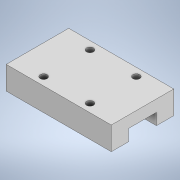
# Autodesk Inventor part: Linear_Rail_Carrier_Basic
Saved by Autodesk Inventor 2021 (Build 250183000, 183)
## iProperties
Created: 2021-03-29
Part Number: Linear_Rail_Carrier_Basic
Material: Generic
Document SubType Name: Modeling
Designer: Ariel Wolle
Density: 1 g/cm^3
Appearance: Default
Author: Ariel Wolle
Autodesk Inventor part; units mm, degrees
ref_plane "YZ Plane" through (0, 0, 0) normal (1, 0, 0) x (0, 1, 0)
ref_plane "XZ Plane" through (0, 0, 0) normal (0, 1, 0) x (-1, 0, 0)
ref_plane "XY Plane" through (0, 0, 0) normal (0, 0, 1) x (1, 0, 0)
sketch "Sketch1" plane through (0, 0, 0) normal (1, 0, 0) x (0, 1, 0)
  line L0 (0, 0) -> (10, 0)
  line L1 (10, 0) -> (10, -27)
  line L2 (10, -27) -> (0, -27)
  line L3 (0, -27) -> (0, 0)
  line L4 (0, -7.5) -> (5, -7.5)
  line L5 (5, -7.5) -> (5, -19.5)
  line L6 (5, -19.5) -> (0, -19.5)
  line L7 (0, -19.5) -> (0, -7.5)
  point P0 (0, -19.5)
  dimension "d0" = 27
  dimension "d1" = 10
  dimension "d2" = 12
  dimension "d3" = 5
  dimension "d4" = 7.5
  constraints: 16 end point, 4 parallel, 2 horizontal, 2 perpendicular, 1 point on line
  measures "d0" distance of L0.end L1.end
  measures "d1" distance of L1.end L2.end
  measures "d2" distance of L4.end L5.end
  measures "d3" distance of L4.start L4.end
  measures "d4" distance between parallel lines of L2 L6
extrude "Extrusion1" add sketch "Sketch1" along normal blind 45.4 contours L0 L1 L2 L3 L6 L5 L4
sketch "Sketch2" plane through (0, 10, 0) normal (0, 1, 0) x (1, 0, 0)
  circle A0 centre (12.7, 3.5) radius 1.5
  circle A1 centre (12.7, 23.5) radius 1.5
  line L0 (0, 0) -> (45.4, 0) projected
  line L1 (0, 27) -> (0, 0) projected
  line L2 (0, 0) -> (45.4, 0) projected
  line L3 (22.7, 0) -> (22.7, 27) construction
  line L4 (0, 27) -> (45.4, 27) projected
  circle A2 centre (32.7, 3.5) radius 1.5
  circle A3 centre (32.7, 23.5) radius 1.5
  dimension "d7" = 20
  dimension "d8" = 3
  dimension "d9" = 3
  dimension "d10" = 3.5
  dimension "d11" = 12.7
  constraints: 4 centre point, 2 end point, 2 midpoint, 2 symmetric about line, 1 vertical alignment, 2 other
  measures "d7" distance of A1.centre A0.centre
  measures "d8" diameter of A0
  measures "d9" diameter of A1
  measures "d10" distance from line of L0 A0.centre
  measures "d11" distance from line of L1 A0.centre
extrude "Extrusion2" cut sketch "Sketch2" against normal blind 45.4
body "Solid1"
